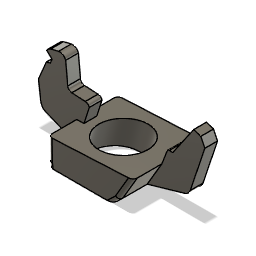
Gel_Blaster_Surge_XL_Front_Tip (Autodesk Fusion 360 design; units mm, degrees)
Autodesk Fusion 360 part; units mm, degrees
note: some values were not read from the file. Set by a fixed rule: which sketch regions a step uses.
sketch "Sketch1" plane through (0, 0, 0) normal (0, 0, 1) x (1, 0, 0)
  line L0 (-26.67, 1.27) -> (-24.1476, 7.2462)
  line L1 (-24.1476, 7.2462) -> (-22.86, 7.62)
  line L2 (-22.86, 7.62) -> (-22.315, 8.9113)
  line L3 (-22.315, 8.9113) -> (-24.003, 10.541)
  line L4 (-23.5873, 11.0942) -> (-22.733, 11.557)
  line L5 (-22.733, 11.557) -> (-20.2207, 12.194)
  arc A0 (-17.9561, 10.8132) -> (-20.2207, 12.194) centre (-19.9, 10.1725) ccw
  arc A1 (-17.272, 4.064) -> (-16.002, 2.794) centre (-16.002, 4.064) ccw
  arc A2 (-10.414, 1.524) -> (-11.684, 2.54) centre (-11.7021, 1.2156) ccw
  line L6 (-16.002, 2.794) -> (-11.684, 2.54)
  line L7 (-17.9561, 10.8132) -> (-17.272, 4.064)
  line L8 (-10.414, 1.524) -> (-12.0756, -3.7274)
  line L9 (-12.0756, -3.7274) -> (12.8223, -2.4887)
  line L10 (12.8223, -2.4887) -> (14.564, 2.0647)
  arc A3 (15.1915, 2.428) -> (14.564, 2.0647) centre (15.0967, 1.8682) ccw
  line L11 (15.1915, 2.428) -> (16.3321, 2.428)
  line L12 (16.3321, 2.428) -> (23.0225, 12.1287)
  line L13 (23.0225, 12.1287) -> (25.292, 11.3722)
  line L14 (25.292, 11.3722) -> (26.5825, 8.7022)
  line L15 (26.5825, 8.7022) -> (21.9101, -5.3151)
  arc A4 (20.1504, -6.9936) -> (21.9101, -5.3151) centre (19.4463, -4.4938) ccw
  arc A5 (-25.9136, -4.4938) -> (-24.2756, -6.6881) centre (-23.4373, -4.3537) ccw
  line L16 (-26.67, 1.27) -> (-25.9136, -4.4938)
  line L17 (-24.2756, -6.6881) -> (-14.3296, -10.6903)
  line L18 (-14.3296, -10.6903) -> (-14.1291, -12.218)
  line L19 (-14.1291, -12.218) -> (6.2698, -12.218)
  line L20 (6.2698, -12.218) -> (8.1283, -10.465)
  line L21 (8.1283, -10.465) -> (20.1504, -6.9936)
  line L22 (-12.0756, -3.7274) -> (-14.4554, -3.8458)
  line L23 (-14.4554, -3.8458) -> (-14.3296, -10.6903)
  line L24 (12.8223, -2.4887) -> (8.1283, -10.465)
  line L25 (-24.003, 10.541) -> (-23.5873, 11.0942)
  constraint parallel L0 L2
  constraint horizontal L11
  constraint perpendicular L13 L15
  constraint tangent L15 A4
  constraint parallel L16 L18
  constraint horizontal L19
  constraint parallel L9 L22
extrude "Extrude1" add sketch "Sketch1" along normal mid plane 4.064 contours L0 L1 L2 L3 L4 L5 A0 A1 A2 L6 L7 L8 A5 L16 L17 L22 L23 L25 | L10 A3 L11 L12 L13 L14 L15 A4 L21 L24 makes body 1 at (-19.0192, -1.7813, 2.032) makes body 2 at (21.6083, 1.9384, 2.032)
extrude "Extrude2" add sketch "Sketch1" along normal mid plane 22.352 contours L9 L18 L19 L20 L22 L23 L24 bodies 1 2
ref_plane "WorkPlane1" through (6.2698, -12.218, 0) normal (0.258819, 0.965926, 0) x (0, 0, 1)
sketch "Sketch4" plane through (6.2698, -12.218, 0) normal (0.258819, 0.965926, 0) x (0, 0, 1)
  line L0 (-11.176, -19.7038) -> (11.176, -19.7038)
  line L1 (-11.176, 0) -> (-11.176, -19.7038) construction
  circle A0 centre (0, -9.8486) radius 7.493
  point P0 (-11.176, 0)
  point P1 (-11.176, 0)
  point P2 (11.176, 0)
  point P3 (0, -9.8486)
  dimension "d6" = 22.352
  dimension "d7" = 19.7038
  dimension "d8" = 9.8552
  dimension "d9" = 11.176
  dimension "d10" = 14.986
  constraint coincident P1 P0
  constraint coincident L0.start L1.end
  constraint coincident P3 A0.centre
  measures "d6" distance of P1 P2
  measures "d7" distance of P0 L0
  measures "d8" distance of L0 P3
  measures "d9" distance of P3 L1
  measures "d10" diameter of A0
extrude "Extrude3" cut sketch "Sketch4" along normal through all and the other way through all bodies 1
fillet "Fillet1" radius 1.27 8 edges at (10.4753, -6.4768, 11.176) (7.1991, -11.3415, 11.176) (-14.3925, -7.268, 11.176) (-14.2293, -11.4541, 11.176) (-14.3925, -7.268, -11.176) (-14.2293, -11.4541, -11.176) (10.4753, -6.4768, -11.176) (7.1991, -11.3415, -11.176) on bodies 1
named bodies: "Surge XL Tip"
